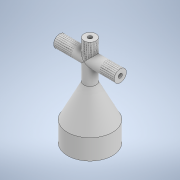
# Autodesk Inventor part: Chemmix
Saved by Autodesk Inventor 2022 (Build 260153070, 153G)
## iProperties
Created: 2021-07-20
Part Number: Chemmix
Material: Generic
Document SubType Name: Modeling
Designer: Eakawit_kor
Density: 1 g/cm^3
Appearance: Default
Author: Eakawit_kor
Autodesk Inventor part; units mm, degrees
ref_plane "YZ Plane" through (0, 0, 0) normal (1, 0, 0) x (0, 1, 0)
ref_plane "XZ Plane" through (0, 0, 0) normal (0, 1, 0) x (-1, 0, 0)
ref_plane "XY Plane" through (0, 0, 0) normal (0, 0, 1) x (1, 0, 0)
sketch "Sketch2" plane through (0, 0, 0) normal (0, 0, 1) x (1, 0, 0)
  line L0 (0, 0) -> (10, 0)
  line L1 (10, 0) -> (0, 20)
  line L2 (0, 20) -> (0, 0)
  line L3 (0, 20) -> (0, 22.2361)
  line L4 (0, 22.2361) -> (11.118, 0)
  line L5 (10, 0) -> (11.118, 0)
  dimension "d4" = 20
  dimension "d8" = 1
  dimension "d9" = 10
  constraints: 12 end point, 2 horizontal, 1 parallel, 1 perpendicular, 1 vertical
  measures "d4" distance of L1.end L0.start
  measures "d8" distance between parallel lines of L4 L1
  measures "d9" distance of L0.start L0.end
revolve "Revolution1" add sketch "Sketch2" angle 360 about axis through (0, 20, 0) along (0, -1, 0) contours L1 L3 L4 L5
sketch "Sketch5" plane through (0, 0, 0) normal (0, -1, 0) x (1, 0, 0)
  circle A0 centre (0, 0) radius 10
  circle A1 centre (0, 0) radius 11.118
  circle A2 centre (0, 0) radius 11.118 projected
  dimension "d11" = 20
  constraints: 2 centre point, 1 coincident, 1 concentric
  measures "d11" diameter of A0
extrude "Extrusion2" add sketch "Sketch5" along normal blind 10
sketch "Sketch7" plane through (0, 0, 0) normal (0, 1, 0) x (-1, 0, 0)
  circle A0 centre (0, 0) radius 1
  dimension "d14" = 2
  constraints: 1 centre point, 1 coincident
  measures "d14" diameter of A0
extrude "Extrusion3" cut sketch "Sketch7" along normal up to surface
sketch "Sketch8" plane through (0, 0, 0) normal (0, 0, 1) x (1, 0, 0)
  line L0 (-1, 20.2361) -> (1, 20.2361) projected
  line L1 (-1, 20.2361) -> (-1, 35.2361)
  line L2 (-1, 35.2361) -> (-3, 35.2361)
  line L3 (-3, 35.2361) -> (-3, 15.9471)
  line L4 (-3, 15.9471) -> (-1, 20.2361)
  line L5 (0, 20.2361) -> (0, 25.2361)
  point P0 (0, 0)
  dimension "d17" = 115
  dimension "d18" = 2
  dimension "d20" = 15
  constraints: 10 end point, 2 perpendicular, 2 vertical, 1 midpoint
  measures "d17" angle of L0 L4
  measures "d18" distance of L1.end L2.end
  measures "d20" distance of L0.start L1.end
revolve "Revolution2" add sketch "Sketch8" angle 360 about axis through (0, 20.2361, 0) along (0, 1, 0)
sketch "Sketch9" plane through (0, 0, 0) normal (1, 0, 0) x (0, 1, 0)
  circle A0 centre (26.2361, 0) radius 3
  line L0 (16.2361, 3) -> (16.2361, -3) projected
  point P0 (0, 0)
  dimension "d22" = 6
  dimension "d23" = 10
  constraints: 1 centre point
  measures "d22" diameter of A0
  measures "d23" distance from line of L0 A0.centre
extrude "Extrusion4" add sketch "Sketch9" along normal mid plane 30
sketch "Sketch10" plane through (-15, 26.2361, 0) normal (-1, 0, 0) x (0, 0, 1)
  circle A0 centre (0, 0) radius 1
  circle A1 centre (0, 0) radius 3 projected
  point P0 (0, -26.2361)
  dimension "d26" = 2
  constraints: 1 centre point, 1 concentric
  measures "d26" diameter of A0
extrude "Extrusion5" cut sketch "Sketch10" against normal up to surface (30 mm away) contours A0
thread "Thread1" size "M6x1" class "6g" standard "ANSI Metric M Profile" length 7.15
thread "Thread2" size "M6x1" class "6g" standard "ANSI Metric M Profile" length 9
thread "Thread3" size "M6x1" class "6g" standard "ANSI Metric M Profile" length 9
sketch "Sketch11" plane through (0, 35.2361, 0) normal (0, 1, 0) x (1, 0, 0)
  circle A0 centre (0, 0) radius 1
  constraints: 1 centre point, 1 coincident
extrude "Extrusion6" cut sketch "Sketch11" against normal blind 20
body "Solid2"
